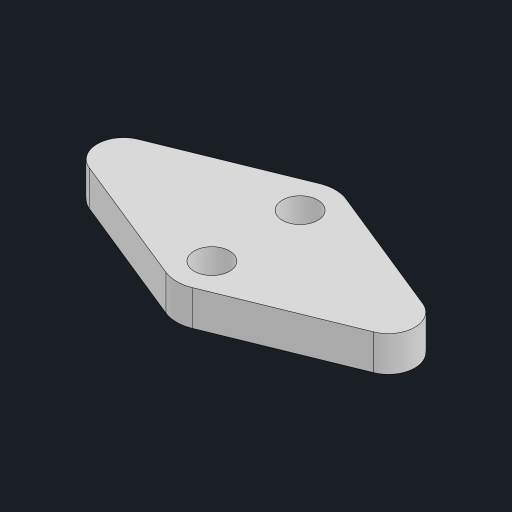
# Autodesk Inventor part: Band_Cap
Saved by Autodesk Inventor 2023 (Build 270158000, 158)
## iProperties
Created: 2022-07-20
Part Number: Band_Cap
Material: 一般
Document SubType Name: Modeling
Designer: legot
Density: 1 g/cm^3
Appearance: 既定
Author: legot
Autodesk Inventor part; units mm, degrees
ref_plane "YZ Plane" through (0, 0, 0) normal (1, 0, 0) x (0, 1, 0)
ref_plane "XZ Plane" through (0, 0, 0) normal (0, 1, 0) x (-1, 0, 0)
ref_plane "XY Plane" through (0, 0, 0) normal (0, 0, 1) x (1, 0, 0)
sketch "スケッチ1" plane through (0, 0, 0) normal (0, 1, 0) x (-1, 0, 0)
  circle A0 centre (7.5, 0) radius 1.5
  circle A1 centre (0, 2.5) radius 2
  circle A2 centre (0, -2.5) radius 2
  circle A3 centre (-7.5, 0) radius 1.5
  line L0 (7.5, 0) -> (-7.5, 0) construction
  line L1 (0, -2.5) -> (0, 2.5) construction
  line L2 (0.7512, 4.3536) -> (8.0634, 1.3902)
  line L3 (8.0634, -1.3902) -> (0.7512, -4.3536)
  line L4 (-0.7512, -4.3536) -> (-8.0634, -1.3902)
  line L5 (-8.0634, 1.3902) -> (-0.7512, 4.3536)
  point P0 (0, 0)
  point P1 (0, 0)
  dimension "d0" = 5
  dimension "d1" = 15
  dimension "d2" = 4
  dimension "d3" = 3
  constraints: 12 end point, 8 point on circle, 8 tangent, 4 centre point, 2 equal radius, 2 midpoint, 1 coincident, 1 horizontal, 1 vertical
  measures "d0" distance of L1.start L1.end
  measures "d1" distance of L0.start L0.end
  measures "d2" diameter of A2
  measures "d3" diameter of A0
extrude "押し出し1" add sketch "スケッチ1" along normal blind 2
sketch "スケッチ2" plane through (0, 2, 0) normal (0, 1, 0) x (1, 0, 0)
  arc A0 (-0.7512, -4.3536) -> (0.7512, -4.3536) centre (0, -2.5) ccw projected
  arc A1 (0.7512, 4.3536) -> (-0.7512, 4.3536) centre (0, 2.5) ccw projected
  point P0 (0, 0)
  constraints: 2 coincident
hole "穴1" at (0, 2, 2.5) at (0, 2, -2.5) direction (0, -1, 0) diameter 2 end through all clearance for "Flat Head Machine Screw (82)" size "#0" standard "Ansi Unified Screw Threads"
